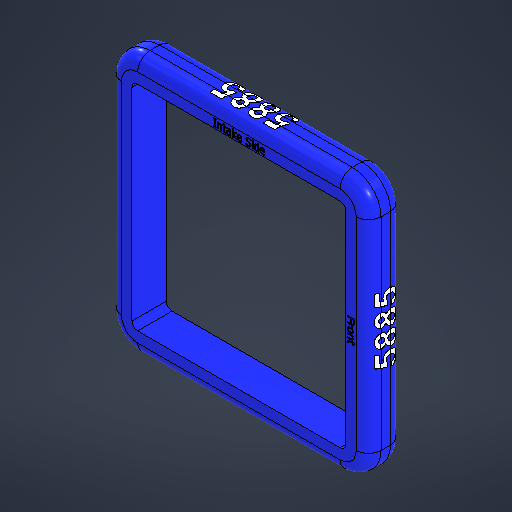
# Autodesk Inventor part: Bumpers
Saved by Autodesk Inventor 2026.1 (Build 301233020, 233B)
## iProperties
Created: 2026-01-21
Part Number: Bumpers
Material: Spruce
Document SubType Name: Modeling
Designer: Jthib
Mass: 13460.1 g
Surface Area: 12229.9 cm^2
Volume: 33650.4 cm^3
Density: 0.4 g/cm^3
Appearance: Blue - Wall Paint - Glossy
Author: Jthib
Autodesk Inventor part; units mm, degrees
ref_plane "YZ Plane" through (0, 0, 0) normal (1, 0, 0) x (0, 1, 0)
ref_plane "XZ Plane" through (0, 0, 0) normal (0, 1, 0) x (-1, 0, 0)
ref_plane "XY Plane" through (0, 0, 0) normal (0, 0, 1) x (1, 0, 0)
sketch "Sketch1" plane through (0, 0, 0) normal (0, 0, 1) x (1, 0, 0)
  line L0 (-349.25, 0) -> (-349.25, 336.55)
  line L1 (-336.55, 349.25) -> (336.55, 349.25)
  line L2 (349.25, 336.55) -> (349.25, -336.55)
  line L3 (336.55, -349.25) -> (-336.55, -349.25)
  line L4 (-349.25, -336.55) -> (-349.25, 0)
  arc A0 (-336.55, 349.25) -> (-349.25, 336.55) centre (-336.55, 336.55) ccw
  arc A1 (349.25, 336.55) -> (336.55, 349.25) centre (336.55, 336.55) ccw
  arc A2 (336.55, -349.25) -> (349.25, -336.55) centre (336.55, -336.55) ccw
  arc A3 (-349.25, -336.55) -> (-336.55, -349.25) centre (-336.55, -336.55) ccw
  point P0 (0, 0)
  point P1 (-349.25, 349.25)
  point P2 (349.25, 349.25)
  point P3 (349.25, -349.25)
  point P4 (-349.25, -349.25)
  dimension "d0" = 698.5
  dimension "d1" = 698.5
  dimension "d2" = 349.25
  dimension "d3" = 349.25
  dimension "d9" = 12.7
  constraints: 10 end point, 9 point on line, 8 point on circle, 8 tangent, 4 centre point, 4 perpendicular, 3 equal radius, 1 collinear, 1 vertical
  measures "d0" distance of point (349.25, 349.25) point (349.25, -349.25)
  measures "d1" distance of point (-349.25, 349.25) point (349.25, 349.25)
  measures "d2" distance from line of point (0, 0) L1
  measures "d3" distance from line of L2 point (0, 0)
  measures "d9" radius of A0
sketch "Sketch2" plane through (0, 0, 0) normal (0, 1, 0) x (-1, 0, 0)
  line L0 (390.525, 61.9125) -> (355.6, 61.9125)
  line L1 (355.6, 61.9125) -> (355.6, -52.3875)
  line L2 (355.6, -52.3875) -> (390.525, -52.3875)
  line L3 (431.8, -11.1125) -> (431.8, 20.6375)
  arc A0 (431.8, 20.6375) -> (390.525, 61.9125) centre (390.525, 20.6375) ccw
  arc A1 (390.525, -52.3875) -> (431.8, -11.1125) centre (390.525, -11.1125) ccw
  line L4 (0, -145.5372) -> (0, 106.4605) construction
  line L5 (355.6, 61.9125) -> (0, 61.9125) construction
  line L6 (355.6, -52.3875) -> (0, -52.3875) construction
  line L7 (-599.1936, -109.5375) -> (599.1891, -109.5375) construction
  point P0 (0, 0)
  point P1 (431.8, 61.9125)
  point P2 (349.25, 0)
  point P3 (349.25, 0)
  point P4 (355.6, 4.7625)
  dimension "d4" = 114.3
  dimension "d5" = 76.2
  dimension "d6" = 41.275
  dimension "d20" = 355.6
  dimension "d21" = 57.15
  constraints: 14 end point, 4 point on circle, 4 point on line, 4 tangent, 3 perpendicular, 2 centre point, 2 horizontal, 2 parallel, 1 equal radius, 1 midpoint, 2 other
  measures "d4" distance of L0.end L1.end
  measures "d5" distance of point (431.8, 61.913) L0.end
  measures "d6" radius of A0
  measures "d20" distance from line of point (0, 0) L1
  measures "d21" distance between parallel lines of L7 L2
sweep "Sweep1" add profiles "Sketch2" path "Sketch1" path curves L0 A0 L1 A1 L2 A2 L3 A3 L4
sketch "Sketch3" plane through (431.8, -336.55, 20.6375) normal (1, 0, 0) x (0, 0, -1)
  line L0 (-23.8125, 82.55) -> (-23.8125, 590.55) construction
  line L1 (-23.8125, 590.55) -> (65.0875, 590.55) construction
  line L2 (65.0875, 590.55) -> (65.0875, 82.55) construction
  line L3 (65.0875, 82.55) -> (-23.8125, 82.55) construction
  line L4 (-23.8125, 82.55) -> (65.0875, 590.55) construction
  line L5 (36.377, 224.9216) -> (35.0992, 239.4995)
  spline S0 degree 2 poles (35.0992, 239.4995) (36.1447, 239.4415) (36.6674, 239.4415) knots 0 0 0 1 1 1
  spline S1 degree 2 poles (36.6674, 239.4415) (41.9526, 239.4415) (47.2378, 244.1459) (47.2378, 247.921) knots 0 0 0 1 2 2 2
  spline S2 degree 2 poles (47.2378, 247.921) (47.2378, 253.2063) (37.132, 261.8601) (28.1878, 261.8601) knots 0 0 0 1 2 2 2
  spline S3 degree 2 poles (28.1878, 261.8601) (22.9026, 261.8601) (17.5012, 256.9814) (17.5012, 252.9159) knots 0 0 0 1 2 2 2
  spline S4 degree 2 poles (17.5012, 252.9159) (17.5012, 250.0119) (20.2309, 244.5524) (22.9607, 241.997) knots 0 0 0 1 2 2 2
  line L6 (22.9607, 241.997) -> (22.0314, 229.7422)
  line L7 (22.0314, 229.7422) -> (-16.9398, 241.3581)
  line L8 (-16.9398, 241.3581) -> (-16.9398, 279.6323)
  line L9 (-16.9398, 279.6323) -> (-3.2912, 276.8445)
  line L10 (-3.2912, 276.8445) -> (-3.2912, 251.522)
  line L11 (-3.2912, 251.522) -> (8.4409, 248.0372)
  spline S5 degree 2 poles (8.4409, 248.0372) (7.4535, 250.2442) (6.4662, 254.6002) (6.4662, 256.7491) knots 0 0 0 1 2 2 2
  spline S6 degree 2 poles (6.4662, 256.7491) (6.4662, 265.461) (18.1982, 276.6703) (28.0716, 276.6703) knots 0 0 0 1 2 2 2
  spline S7 degree 2 poles (28.0716, 276.6703) (35.9704, 276.6703) (51.3034, 268.8296) (59.4925, 254.8906) (59.4925, 247.2822) knots 0 0 0 1 2 3 3 3
  spline S8 degree 2 poles (59.4925, 247.2822) (59.4925, 237.5249) (46.9474, 225.0378) (36.377, 224.9216) knots 0 0 0 1 2 2 2
  spline S9 degree 2 poles (16.2816, 300.2505) (13.668, 296.243) (6.6985, 292.2355) (2.5168, 292.2355) knots 0 0 0 1 2 2 2
  spline S10 degree 2 poles (2.5168, 292.2355) (-2.42, 292.2355) (-12.5258, 297.8692) (-18.3337, 309.0204) (-18.3337, 316.1061) knots 0 0 0 1 2 3 3 3
  spline S11 degree 2 poles (-18.3337, 316.1061) (-18.3337, 326.27) (-7.7052, 337.7116) (0.4259, 337.7116) knots 0 0 0 1 2 2 2
  spline S12 degree 2 poles (0.4259, 337.7116) (6.1177, 337.7116) (14.6553, 331.2648) (17.4431, 324.818) knots 0 0 0 1 2 2 2
  spline S13 degree 2 poles (17.4431, 324.818) (20.289, 329.4643) (28.4782, 334.1107) (33.7053, 334.1107) knots 0 0 0 1 2 2 2
  spline S14 degree 2 poles (33.7053, 334.1107) (42.3591, 334.1107) (49.4448, 328.5931) knots 0 0 0 1 1 1
  spline S15 degree 2 poles (49.4448, 328.5931) (59.6087, 320.5782) (59.6087, 306.7553) knots 0 0 0 1 1 1
  spline S16 degree 2 poles (59.6087, 306.7553) (59.6087, 296.6495) (47.7024, 284.3948) (38.5259, 284.3948) knots 0 0 0 1 2 2 2
  spline S17 degree 2 poles (38.5259, 284.3948) (30.8595, 284.3948) (18.779, 292.9325) (16.2816, 300.2505) knots 0 0 0 1 2 2 2
  spline S18 degree 2 poles (38.7582, 299.2631) (43.0561, 299.2631) (47.9348, 303.9095) (47.9348, 307.6846) knots 0 0 0 1 2 2 2
  spline S19 degree 2 poles (47.9348, 307.6846) (47.9348, 313.4345) (37.7128, 319.707) (31.7306, 319.707) knots 0 0 0 1 2 2 2
  spline S20 degree 2 poles (31.7306, 319.707) (27.8974, 319.707) (22.9607, 314.8864) (22.9607, 311.1694) knots 0 0 0 1 2 2 2
  spline S21 degree 2 poles (22.9607, 311.1694) (22.9607, 306.4649) (31.6145, 299.2631) (38.7582, 299.2631) knots 0 0 0 1 2 2 2
  spline S22 degree 2 poles (3.5041, 305.8841) (7.105, 305.8841) (11.5191, 310.2401) (11.5191, 313.7248) knots 0 0 0 1 2 2 2
  spline S23 degree 2 poles (11.5191, 313.7248) (11.5191, 317.7323) (5.4207, 323.8306) (1.3552, 323.8306) knots 0 0 0 1 2 2 2
  spline S24 degree 2 poles (1.3552, 323.8306) (-2.3038, 323.8306) (-6.8921, 319.3585) (-6.8921, 315.8738) knots 0 0 0 1 2 2 2
  spline S25 degree 2 poles (-6.8921, 315.8738) (-6.8921, 311.7502) (-0.8518, 305.8841) (3.5041, 305.8841) knots 0 0 0 1 2 2 2
  spline S26 degree 2 poles (16.2816, 359.4332) (13.668, 355.4258) (6.6985, 351.4183) (2.5168, 351.4183) knots 0 0 0 1 2 2 2
  spline S27 degree 2 poles (2.5168, 351.4183) (-2.42, 351.4183) (-12.5258, 357.052) (-18.3337, 368.2032) (-18.3337, 375.2889) knots 0 0 0 1 2 3 3 3
  spline S28 degree 2 poles (-18.3337, 375.2889) (-18.3337, 385.4527) (-7.7052, 396.8944) (0.4259, 396.8944) knots 0 0 0 1 2 2 2
  spline S29 degree 2 poles (0.4259, 396.8944) (6.1177, 396.8944) (14.6553, 390.4476) (17.4431, 384.0008) knots 0 0 0 1 2 2 2
  spline S30 degree 2 poles (17.4431, 384.0008) (20.289, 388.6471) (28.4782, 393.2934) (33.7053, 393.2934) knots 0 0 0 1 2 2 2
  spline S31 degree 2 poles (33.7053, 393.2934) (42.3591, 393.2934) (49.4448, 387.7759) knots 0 0 0 1 1 1
  spline S32 degree 2 poles (49.4448, 387.7759) (59.6087, 379.761) (59.6087, 365.9381) knots 0 0 0 1 1 1
  spline S33 degree 2 poles (59.6087, 365.9381) (59.6087, 355.8323) (47.7024, 343.5776) (38.5259, 343.5776) knots 0 0 0 1 2 2 2
  spline S34 degree 2 poles (38.5259, 343.5776) (30.8595, 343.5776) (18.779, 352.1152) (16.2816, 359.4332) knots 0 0 0 1 2 2 2
  spline S35 degree 2 poles (38.7582, 358.4459) (43.0561, 358.4459) (47.9348, 363.0922) (47.9348, 366.8674) knots 0 0 0 1 2 2 2
  spline S36 degree 2 poles (47.9348, 366.8674) (47.9348, 372.6172) (37.7128, 378.8898) (31.7306, 378.8898) knots 0 0 0 1 2 2 2
  spline S37 degree 2 poles (31.7306, 378.8898) (27.8974, 378.8898) (22.9607, 374.0692) (22.9607, 370.3521) knots 0 0 0 1 2 2 2
  spline S38 degree 2 poles (22.9607, 370.3521) (22.9607, 365.6477) (31.6145, 358.4459) (38.7582, 358.4459) knots 0 0 0 1 2 2 2
  spline S39 degree 2 poles (3.5041, 365.0669) (7.105, 365.0669) (11.5191, 369.4229) (11.5191, 372.9076) knots 0 0 0 1 2 2 2
  spline S40 degree 2 poles (11.5191, 372.9076) (11.5191, 376.9151) (5.4207, 383.0134) (1.3552, 383.0134) knots 0 0 0 1 2 2 2
  spline S41 degree 2 poles (1.3552, 383.0134) (-2.3038, 383.0134) (-6.8921, 378.5413) (-6.8921, 375.0566) knots 0 0 0 1 2 2 2
  spline S42 degree 2 poles (-6.8921, 375.0566) (-6.8921, 370.9329) (-0.8518, 365.0669) (3.5041, 365.0669) knots 0 0 0 1 2 2 2
  line L12 (36.377, 402.47) -> (35.0992, 417.0479)
  spline S43 degree 2 poles (35.0992, 417.0479) (36.1447, 416.9898) (36.6674, 416.9898) knots 0 0 0 1 1 1
  spline S44 degree 2 poles (36.6674, 416.9898) (41.9526, 416.9898) (47.2378, 421.6942) (47.2378, 425.4694) knots 0 0 0 1 2 2 2
  spline S45 degree 2 poles (47.2378, 425.4694) (47.2378, 430.7546) (37.132, 439.4084) (28.1878, 439.4084) knots 0 0 0 1 2 2 2
  spline S46 degree 2 poles (28.1878, 439.4084) (22.9026, 439.4084) (17.5012, 434.5297) (17.5012, 430.4642) knots 0 0 0 1 2 2 2
  spline S47 degree 2 poles (17.5012, 430.4642) (17.5012, 427.5602) (20.2309, 422.1008) (22.9607, 419.5453) knots 0 0 0 1 2 2 2
  line L13 (22.9607, 419.5453) -> (22.0314, 407.2905)
  line L14 (22.0314, 407.2905) -> (-16.9398, 418.9064)
  line L15 (-16.9398, 418.9064) -> (-16.9398, 457.1806)
  line L16 (-16.9398, 457.1806) -> (-3.2912, 454.3928)
  line L17 (-3.2912, 454.3928) -> (-3.2912, 429.0703)
  line L18 (-3.2912, 429.0703) -> (8.4409, 425.5855)
  spline S48 degree 2 poles (8.4409, 425.5855) (7.4535, 427.7925) (6.4662, 432.1485) (6.4662, 434.2974) knots 0 0 0 1 2 2 2
  spline S49 degree 2 poles (6.4662, 434.2974) (6.4662, 443.0093) (18.1982, 454.2186) (28.0716, 454.2186) knots 0 0 0 1 2 2 2
  spline S50 degree 2 poles (28.0716, 454.2186) (35.9704, 454.2186) (51.3034, 446.3779) (59.4925, 432.4389) (59.4925, 424.8305) knots 0 0 0 1 2 3 3 3
  spline S51 degree 2 poles (59.4925, 424.8305) (59.4925, 415.0732) (46.9474, 402.5861) (36.377, 402.47) knots 0 0 0 1 2 2 2
  point P0 (20.6375, 336.55)
  point P1 (20.6375, 336.55)
  dimension "d2" = 349.25
  dimension "d10" = 508
  dimension "d11" = 88.9
  constraints: 2 end point, 1 coincident, 1 horizontal, 1 midpoint, 2 other
  measures "d10" distance of L0.start L0.end
  measures "d11" distance of L0.end L1.end
emboss "Emboss1" sketch "Sketch3" operation cut depth 0.254 direction (-1, 0, 0)
pattern_circular "Circular Pattern1" count 4 over 360 about axis through (0, 0, -10) along (0, 0, 1) of "Emboss1"
sketch "Sketch4" plane through (-336.55, -390.525, 61.9125) normal (0, 0, 1) x (1, 0, 0)
  line L0 (692.15, 517.525) -> (692.15, 263.525) construction
  line L1 (692.15, 263.525) -> (727.075, 263.525) construction
  line L2 (727.075, 263.525) -> (727.075, 517.525) construction
  line L3 (727.075, 517.525) -> (692.15, 517.525) construction
  line L4 (692.15, 727.075) -> (692.15, 53.975) projected
  line L5 (727.075, 727.075) -> (727.075, 53.975) projected
  line L6 (719.5749, 413.2286) -> (719.5749, 425.0435)
  line L7 (719.5749, 425.0435) -> (712.4119, 425.0435)
  line L8 (712.4119, 425.0435) -> (712.4119, 413.7226)
  line L9 (712.4119, 413.7226) -> (709.4067, 413.7226)
  line L10 (709.4067, 413.7226) -> (709.4067, 425.0435)
  line L11 (709.4067, 425.0435) -> (697.1801, 425.0435)
  line L12 (697.1801, 425.0435) -> (697.1801, 428.4192)
  line L13 (697.1801, 428.4192) -> (722.5801, 428.4192)
  line L14 (722.5801, 428.4192) -> (722.5801, 413.2286)
  line L15 (722.5801, 413.2286) -> (719.5749, 413.2286)
  line L16 (712.8029, 400.3433) -> (712.8029, 400.508)
  spline S0 degree 2 poles (712.8029, 400.508) (712.9059, 400.8785) (712.947, 401.6812) (712.947, 402.237) knots 0 0 0 1 2 2 2
  spline S1 degree 2 poles (712.947, 402.237) (712.947, 403.5337) (711.8149, 406.0861) (710.7034, 407.2388) knots 0 0 0 1 2 2 2
  line L17 (710.7034, 407.2388) -> (697.1801, 407.2388)
  line L18 (697.1801, 407.2388) -> (697.1801, 410.4498)
  line L19 (697.1801, 410.4498) -> (716.2404, 410.4498)
  line L20 (716.2404, 410.4498) -> (716.2404, 407.2388)
  line L21 (716.2404, 407.2388) -> (713.3999, 407.2388)
  spline S2 degree 2 poles (713.3999, 407.2388) (714.9642, 405.4892) (716.2404, 402.8751) (716.2404, 401.6401) knots 0 0 0 1 2 2 2
  spline S3 degree 2 poles (716.2404, 401.6401) (716.2404, 401.1461) (716.1992, 400.6521) (716.1375, 400.3433) knots 0 0 0 1 2 2 2
  line L22 (716.1375, 400.3433) -> (712.8029, 400.3433)
  spline S4 degree 2 poles (706.7102, 382.1887) (701.8937, 382.1887) (696.6449, 386.82) (696.6449, 390.6897) knots 0 0 0 1 2 2 2
  spline S5 degree 2 poles (696.6449, 390.6897) (696.6449, 394.6623) (702.0584, 399.2112) (706.7102, 399.2112) knots 0 0 0 1 2 2 2
  spline S6 degree 2 poles (706.7102, 399.2112) (711.4856, 399.2112) (716.7755, 394.5182) (716.7755, 390.6897) knots 0 0 0 1 2 2 2
  spline S7 degree 2 poles (716.7755, 390.6897) (716.7755, 386.82) (711.5062, 382.1887) (706.7102, 382.1887) knots 0 0 0 1 2 2 2
  spline S8 degree 2 poles (706.7102, 385.5026) (710.4153, 385.5026) (714.0174, 388.1991) (714.0174, 390.6897) knots 0 0 0 1 2 2 2
  spline S9 degree 2 poles (714.0174, 390.6897) (714.0174, 393.1803) (710.4153, 395.8973) (706.7102, 395.8973) knots 0 0 0 1 2 2 2
  spline S10 degree 2 poles (706.7102, 395.8973) (703.1081, 395.8973) (699.4031, 393.1803) (699.4031, 390.6897) knots 0 0 0 1 2 2 2
  spline S11 degree 2 poles (699.4031, 390.6897) (699.4031, 388.2196) (703.0464, 385.5026) (706.7102, 385.5026) knots 0 0 0 1 2 2 2
  line L23 (697.1801, 363.9312) -> (697.1801, 367.1422)
  line L24 (697.1801, 367.1422) -> (708.0482, 367.1422)
  spline S12 degree 2 poles (708.0482, 367.1422) (709.3655, 367.1422) (711.6297, 367.3892) (712.3089, 367.7597) knots 0 0 0 1 2 2 2
  spline S13 degree 2 poles (712.3089, 367.7597) (713.0294, 368.1508) (713.7292, 369.5504) (713.7292, 370.7443) knots 0 0 0 1 2 2 2
  spline S14 degree 2 poles (713.7292, 370.7443) (713.7292, 371.9381) (712.453, 374.4699) (711.4238, 375.6843) knots 0 0 0 1 2 2 2
  line L25 (711.4238, 375.6843) -> (697.1801, 375.6843)
  line L26 (697.1801, 375.6843) -> (697.1801, 378.8953)
  line L27 (697.1801, 378.8953) -> (716.2404, 378.8953)
  line L28 (716.2404, 378.8953) -> (716.2404, 375.6843)
  line L29 (716.2404, 375.6843) -> (714.1203, 375.6843)
  spline S15 degree 2 poles (714.1203, 375.6843) (715.417, 374.2435) (716.7755, 371.4647) (716.7755, 369.9004) knots 0 0 0 1 2 2 2
  spline S16 degree 2 poles (716.7755, 369.9004) (716.7755, 367.101) (713.0705, 363.9312) (709.5507, 363.9312) knots 0 0 0 1 2 2 2
  line L30 (709.5507, 363.9312) -> (697.1801, 363.9312)
  spline S17 degree 2 poles (696.8096, 353.66) (696.8096, 356.2741) (699.7942, 359.2175) (703.0258, 359.2175) knots 0 0 0 1 2 2 2
  line L31 (703.0258, 359.2175) -> (713.5851, 359.2175)
  line L32 (713.5851, 359.2175) -> (713.5851, 361.3788)
  line L33 (713.5851, 361.3788) -> (716.2404, 361.3788)
  line L34 (716.2404, 361.3788) -> (716.2404, 359.2175)
  line L35 (716.2404, 359.2175) -> (721.7156, 359.2175)
  line L36 (721.7156, 359.2175) -> (721.7156, 356.0065)
  line L37 (721.7156, 356.0065) -> (716.2404, 356.0065)
  line L38 (716.2404, 356.0065) -> (716.2404, 350.0991)
  line L39 (716.2404, 350.0991) -> (713.5851, 350.0991)
  line L40 (713.5851, 350.0991) -> (713.5851, 356.0065)
  line L41 (713.5851, 356.0065) -> (704.5078, 356.0065)
  spline S18 degree 2 poles (704.5078, 356.0065) (703.067, 356.0065) (701.482, 355.9036) (700.8028, 355.5537) knots 0 0 0 1 2 2 2
  spline S19 degree 2 poles (700.8028, 355.5537) (700.2059, 355.2655) (699.6089, 353.9688) (699.6089, 352.8573) knots 0 0 0 1 2 2 2
  spline S20 degree 2 poles (699.6089, 352.8573) (699.6089, 352.0751) (700.0824, 350.6137) (700.2264, 350.2843) knots 0 0 0 1 2 2 2
  line L42 (700.2264, 350.2843) -> (700.2264, 350.0991)
  line L43 (700.2264, 350.0991) -> (697.3448, 350.0991)
  spline S21 degree 2 poles (697.3448, 350.0991) (697.0978, 351.0047) (696.8096, 352.8573) (696.8096, 353.66) knots 0 0 0 1 2 2 2
  point P0 (336.55, 390.525)
  point P1 (727.075, 390.525)
  dimension "d2" = 349.25
  dimension "d17" = 254
  constraints: 2 midpoint, 1 collinear, 2 other
  measures "d17" distance between parallel lines of L1 L3
emboss "Emboss2" sketch "Sketch4" operation cut depth 0.254 direction (0, 0, -1)
sketch "Sketch5" plane through (-336.55, -390.525, 61.9125) normal (0, 0, 1) x (1, 0, 0)
  line L0 (0, 781.05) -> (673.1, 781.05) construction
  line L1 (673.1, 781.05) -> (673.1, 746.125) construction
  line L2 (673.1, 746.125) -> (0, 746.125) construction
  line L3 (0, 746.125) -> (0, 781.05) construction
  line L4 (0, 781.05) -> (673.1, 781.05) construction
  line L5 (0, 746.125) -> (673.1, 746.125) construction
  line L6 (336.55, -215.9) -> (336.55, 1006.475) construction
  line L7 (260.8028, 750.589) -> (250.9639, 750.589)
  line L8 (250.9639, 750.589) -> (250.9639, 753.1826)
  line L9 (250.9639, 753.1826) -> (254.1955, 753.1826)
  line L10 (254.1955, 753.1826) -> (254.1955, 773.3955)
  line L11 (254.1955, 773.3955) -> (250.9639, 773.3955)
  line L12 (250.9639, 773.3955) -> (250.9639, 775.989)
  line L13 (250.9639, 775.989) -> (260.8028, 775.989)
  line L14 (260.8028, 775.989) -> (260.8028, 773.3955)
  line L15 (260.8028, 773.3955) -> (257.5712, 773.3955)
  line L16 (257.5712, 773.3955) -> (257.5712, 753.1826)
  line L17 (257.5712, 753.1826) -> (260.8028, 753.1826)
  line L18 (260.8028, 753.1826) -> (260.8028, 750.589)
  line L19 (279.6985, 750.589) -> (276.4874, 750.589)
  line L20 (276.4874, 750.589) -> (276.4874, 761.4571)
  spline S0 degree 2 poles (276.4874, 761.4571) (276.4874, 762.7745) (276.2404, 765.0386) (275.8699, 765.7179) knots 0 0 0 1 2 2 2
  spline S1 degree 2 poles (275.8699, 765.7179) (275.4789, 766.4383) (274.0792, 767.1381) (272.8853, 767.1381) knots 0 0 0 1 2 2 2
  spline S2 degree 2 poles (272.8853, 767.1381) (271.6915, 767.1381) (269.1597, 765.862) (267.9453, 764.8328) knots 0 0 0 1 2 2 2
  line L21 (267.9453, 764.8328) -> (267.9453, 750.589)
  line L22 (267.9453, 750.589) -> (264.7343, 750.589)
  line L23 (264.7343, 750.589) -> (264.7343, 769.6493)
  line L24 (264.7343, 769.6493) -> (267.9453, 769.6493)
  line L25 (267.9453, 769.6493) -> (267.9453, 767.5292)
  spline S3 degree 2 poles (267.9453, 767.5292) (269.3861, 768.826) (272.1649, 770.1845) (273.7293, 770.1845) knots 0 0 0 1 2 2 2
  spline S4 degree 2 poles (273.7293, 770.1845) (276.5286, 770.1845) (279.6985, 766.4795) (279.6985, 762.9597) knots 0 0 0 1 2 2 2
  line L26 (279.6985, 762.9597) -> (279.6985, 750.589)
  spline S5 degree 2 poles (289.9696, 750.2185) (287.3555, 750.2185) (284.4121, 753.2031) (284.4121, 756.4347) knots 0 0 0 1 2 2 2
  line L27 (284.4121, 756.4347) -> (284.4121, 766.9941)
  line L28 (284.4121, 766.9941) -> (282.2508, 766.9941)
  line L29 (282.2508, 766.9941) -> (282.2508, 769.6493)
  line L30 (282.2508, 769.6493) -> (284.4121, 769.6493)
  line L31 (284.4121, 769.6493) -> (284.4121, 775.1245)
  line L32 (284.4121, 775.1245) -> (287.6231, 775.1245)
  line L33 (287.6231, 775.1245) -> (287.6231, 769.6493)
  line L34 (287.6231, 769.6493) -> (293.5306, 769.6493)
  line L35 (293.5306, 769.6493) -> (293.5306, 766.9941)
  line L36 (293.5306, 766.9941) -> (287.6231, 766.9941)
  line L37 (287.6231, 766.9941) -> (287.6231, 757.9168)
  spline S6 degree 2 poles (287.6231, 757.9168) (287.6231, 756.4759) (287.726, 754.891) (288.0759, 754.2117) knots 0 0 0 1 2 2 2
  spline S7 degree 2 poles (288.0759, 754.2117) (288.3641, 753.6148) (289.6609, 753.0179) (290.7724, 753.0179) knots 0 0 0 1 2 2 2
  spline S8 degree 2 poles (290.7724, 753.0179) (291.5545, 753.0179) (293.016, 753.4913) (293.3453, 753.6354) knots 0 0 0 1 2 2 2
  line L38 (293.3453, 753.6354) -> (293.5306, 753.6354)
  line L39 (293.5306, 753.6354) -> (293.5306, 750.7537)
  spline S9 degree 2 poles (293.5306, 750.7537) (292.6249, 750.5067) (290.7724, 750.2185) (289.9696, 750.2185) knots 0 0 0 1 2 2 2
  spline S10 degree 2 poles (306.5187, 752.6062) (306.1276, 752.3181) (304.8103, 751.2889) (304.1928, 750.9801) knots 0 0 0 1 2 2 2
  spline S11 degree 2 poles (304.1928, 750.9801) (303.3489, 750.5273) (301.7639, 750.0539) (300.3231, 750.0539) knots 0 0 0 1 2 2 2
  spline S12 degree 2 poles (300.3231, 750.0539) (299.1498, 750.0539) (297.0297, 750.939) (296.227, 751.7417) knots 0 0 0 1 2 2 2
  spline S13 degree 2 poles (296.227, 751.7417) (295.4654, 752.5239) (294.5391, 754.8292) (294.5391, 756.1054) knots 0 0 0 1 2 2 2
  spline S14 degree 2 poles (294.5391, 756.1054) (294.5391, 758.0814) (296.2064, 760.8808) (298.0178, 761.6835) knots 0 0 0 1 2 2 2
  spline S15 degree 2 poles (298.0178, 761.6835) (299.6233, 762.4245) (303.987, 762.9803) (306.5187, 763.1244) knots 0 0 0 1 2 2 2
  line L40 (306.5187, 763.1244) -> (306.5187, 763.7419)
  spline S16 degree 2 poles (306.5187, 763.7419) (306.5187, 764.8534) (305.8395, 766.2325) (305.222, 766.6236) knots 0 0 0 1 2 2 2
  spline S17 degree 2 poles (305.222, 766.6236) (304.6045, 767.0146) (302.8343, 767.2616) (301.8874, 767.2616) knots 0 0 0 1 2 2 2
  spline S18 degree 2 poles (301.8874, 767.2616) (300.7759, 767.2616) (297.7708, 766.603) (296.2682, 765.9649) knots 0 0 0 1 2 2 2
  line L41 (296.2682, 765.9649) -> (296.0829, 765.9649)
  line L42 (296.0829, 765.9649) -> (296.0829, 769.2377)
  spline S19 degree 2 poles (296.0829, 769.2377) (296.968, 769.4847) (300.2819, 770.1022) (301.908, 770.1022) knots 0 0 0 1 2 2 2
  spline S20 degree 2 poles (301.908, 770.1022) (303.884, 770.1022) (306.5805, 769.4847) (307.6508, 768.6819) knots 0 0 0 1 2 2 2
  spline S21 degree 2 poles (307.6508, 768.6819) (308.7006, 767.8997) (309.7297, 765.4091) (309.7297, 763.6184) knots 0 0 0 1 2 2 2
  line L43 (309.7297, 763.6184) -> (309.7297, 750.589)
  line L44 (309.7297, 750.589) -> (306.5187, 750.589)
  line L45 (306.5187, 750.589) -> (306.5187, 752.6062)
  line L46 (306.5187, 755.2821) -> (306.5187, 760.572)
  spline S22 degree 2 poles (306.5187, 760.572) (305.3661, 760.4691) (301.8874, 760.1192) (300.7965, 759.7899) knots 0 0 0 1 2 2 2
  spline S23 degree 2 poles (300.7965, 759.7899) (299.5203, 759.3988) (297.8531, 757.7727) (297.8531, 756.3318) knots 0 0 0 1 2 2 2
  spline S24 degree 2 poles (297.8531, 756.3318) (297.8531, 754.6852) (299.7056, 753.0179) (301.4758, 753.0179) knots 0 0 0 1 2 2 2
  spline S25 degree 2 poles (301.4758, 753.0179) (302.9784, 753.0179) (305.4484, 754.3146) (306.5187, 755.2821) knots 0 0 0 1 2 2 2
  line L47 (330.025, 750.589) -> (325.8054, 750.589)
  line L48 (325.8054, 750.589) -> (318.7247, 759.7899)
  line L49 (318.7247, 759.7899) -> (317.4485, 758.5548)
  line L50 (317.4485, 758.5548) -> (317.4485, 750.589)
  line L51 (317.4485, 750.589) -> (314.2375, 750.589)
  line L52 (314.2375, 750.589) -> (314.2375, 777.1211)
  line L53 (314.2375, 777.1211) -> (317.4485, 777.1211)
  line L54 (317.4485, 777.1211) -> (317.4485, 761.6012)
  line L55 (317.4485, 761.6012) -> (324.9821, 769.6493)
  line L56 (324.9821, 769.6493) -> (328.9753, 769.6493)
  line L57 (328.9753, 769.6493) -> (321.1536, 761.6835)
  line L58 (321.1536, 761.6835) -> (330.025, 750.589)
  spline S26 degree 2 poles (339.9051, 750.1568) (335.3356, 750.1568) (330.3132, 755.2821) (330.3132, 760.0163) knots 0 0 0 1 2 2 2
  spline S27 degree 2 poles (330.3132, 760.0163) (330.3132, 764.6681) (335.1915, 770.1845) (339.1229, 770.1845) knots 0 0 0 1 2 2 2
  spline S28 degree 2 poles (339.1229, 770.1845) (340.8931, 770.1845) (343.6307, 769.1553) (344.6393, 768.0644) knots 0 0 0 1 2 2 2
  spline S29 degree 2 poles (344.6393, 768.0644) (345.6685, 766.9735) (346.7594, 763.8242) (346.7594, 761.5394) knots 0 0 0 1 2 2 2
  line L59 (346.7594, 761.5394) -> (346.7594, 759.7899)
  line L60 (346.7594, 759.7899) -> (333.5654, 759.7899)
  spline S30 degree 2 poles (333.5654, 759.7899) (333.5654, 756.4759) (336.8999, 752.9561) (339.8639, 752.9561) knots 0 0 0 1 2 2 2
  spline S31 degree 2 poles (339.8639, 752.9561) (340.9137, 752.9561) (342.9515, 753.4296) (343.7748, 753.8001) knots 0 0 0 1 2 2 2
  spline S32 degree 2 poles (343.7748, 753.8001) (344.6393, 754.2117) (345.8331, 754.9322) (346.2242, 755.2615) knots 0 0 0 1 2 2 2
  line L61 (346.2242, 755.2615) -> (346.4095, 755.2615)
  line L62 (346.4095, 755.2615) -> (346.4095, 751.7623)
  spline S33 degree 2 poles (346.4095, 751.7623) (345.8537, 751.5359) (344.1659, 750.8772) (343.5072, 750.692) knots 0 0 0 1 2 2 2
  spline S34 degree 2 poles (343.5072, 750.692) (342.581, 750.4244) (341.0578, 750.1568) (339.9051, 750.1568) knots 0 0 0 1 2 2 2
  spline S35 degree 2 poles (343.6307, 762.2393) (343.5896, 763.536) (343.0544, 765.4297) (342.5398, 766.0678) knots 0 0 0 1 2 2 2
  spline S36 degree 2 poles (342.5398, 766.0678) (341.984, 766.7882) (340.2344, 767.5498) (338.9377, 767.5498) knots 0 0 0 1 2 2 2
  spline S37 degree 2 poles (338.9377, 767.5498) (337.6615, 767.5498) (335.8708, 766.7882) (335.1297, 766.0472) knots 0 0 0 1 2 2 2
  spline S38 degree 2 poles (335.1297, 766.0472) (334.4093, 765.2856) (333.6683, 763.4537) (333.5654, 762.2393) knots 0 0 0 1 2 2 2
  line L63 (333.5654, 762.2393) -> (343.6307, 762.2393)
  spline S39 degree 2 poles (368.2485, 750.1362) (365.4904, 750.1362) (361.6207, 751.2889) (359.9122, 752.1122) knots 0 0 0 1 2 2 2
  line L64 (359.9122, 752.1122) -> (359.9122, 756.3524)
  line L65 (359.9122, 756.3524) -> (360.1592, 756.3524)
  spline S40 degree 2 poles (360.1592, 756.3524) (361.8265, 754.7881) (366.0461, 753.0591) (368.0015, 753.0591) knots 0 0 0 1 2 2 2
  spline S41 degree 2 poles (368.0015, 753.0591) (370.8009, 753.0591) (373.662, 755.385) (373.662, 757.2993) knots 0 0 0 1 2 2 2
  spline S42 degree 2 poles (373.662, 757.2993) (373.662, 758.8224) (372.1594, 760.7161) (370.5333, 761.1895) knots 0 0 0 1 2 2 2
  spline S43 degree 2 poles (370.5333, 761.1895) (369.3601, 761.5189) (367.4046, 761.9717) (365.9432, 762.3422) knots 0 0 0 1 2 2 2
  spline S44 degree 2 poles (365.9432, 762.3422) (364.6259, 762.6921) (362.5469, 763.7419) (361.7442, 764.5858) knots 0 0 0 1 2 2 2
  spline S45 degree 2 poles (361.7442, 764.5858) (360.962, 765.4297) (360.0975, 767.6939) (360.0975, 769.1759) knots 0 0 0 1 2 2 2
  spline S46 degree 2 poles (360.0975, 769.1759) (360.0975, 772.2634) (364.914, 776.4419) (368.6396, 776.4419) knots 0 0 0 1 2 2 2
  spline S47 degree 2 poles (368.6396, 776.4419) (370.7803, 776.4419) (374.5677, 775.598) (376.1938, 774.7952) knots 0 0 0 1 2 2 2
  line L66 (376.1938, 774.7952) -> (376.1938, 770.7608)
  line L67 (376.1938, 770.7608) -> (375.9468, 770.7608)
  spline S48 degree 2 poles (375.9468, 770.7608) (374.7323, 771.8723) (370.945, 773.519) (368.866, 773.519) knots 0 0 0 1 2 2 2
  spline S49 degree 2 poles (368.866, 773.519) (366.5195, 773.519) (363.6173, 771.3166) (363.6173, 769.5258) knots 0 0 0 1 2 2 2
  spline S50 degree 2 poles (363.6173, 769.5258) (363.6173, 767.9203) (365.3257, 766.0061) (366.9312, 765.5738) knots 0 0 0 1 2 2 2
  spline S51 degree 2 poles (366.9312, 765.5738) (368.0015, 765.2856) (371.1096, 764.5446) (372.1388, 764.2359) knots 0 0 0 1 2 2 2
  spline S52 degree 2 poles (372.1388, 764.2359) (374.7529, 763.4331) (377.1818, 760.2015) (377.1818, 757.8344) knots 0 0 0 1 2 2 2
  spline S53 degree 2 poles (377.1818, 757.8344) (377.1818, 756.3318) (375.9673, 753.4501) (374.8764, 752.4416) knots 0 0 0 1 2 2 2
  spline S54 degree 2 poles (374.8764, 752.4416) (373.662, 751.33) (370.5745, 750.1362) (368.2485, 750.1362) knots 0 0 0 1 2 2 2
  line L68 (383.645, 750.589) -> (380.434, 750.589)
  line L69 (380.434, 750.589) -> (380.434, 769.6493)
  line L70 (380.434, 769.6493) -> (383.645, 769.6493)
  line L71 (383.645, 769.6493) -> (383.645, 750.589)
  line L72 (383.8714, 772.8192) -> (380.2281, 772.8192)
  line L73 (380.2281, 772.8192) -> (380.2281, 776.1537)
  line L74 (380.2281, 776.1537) -> (383.8714, 776.1537)
  line L75 (383.8714, 776.1537) -> (383.8714, 772.8192)
  line L76 (403.014, 750.589) -> (399.803, 750.589)
  line L77 (399.803, 750.589) -> (399.803, 752.5239)
  spline S55 degree 2 poles (399.803, 752.5239) (399.062, 751.9064) (397.9711, 751.083) (397.2301, 750.7331) knots 0 0 0 1 2 2 2
  spline S56 degree 2 poles (397.2301, 750.7331) (396.5508, 750.4038) (395.0894, 750.0539) (394.122, 750.0539) knots 0 0 0 1 2 2 2
  spline S57 degree 2 poles (394.122, 750.0539) (392.5576, 750.0539) (389.9229, 751.3506) (388.9967, 752.6062) knots 0 0 0 1 2 2 2
  spline S58 degree 2 poles (388.9967, 752.6062) (388.0704, 753.8618) (387.0413, 757.5668) (387.0413, 759.9751) knots 0 0 0 1 2 2 2
  spline S59 degree 2 poles (387.0413, 759.9751) (387.0413, 762.4863) (388.338, 766.1501) (389.4701, 767.5292) knots 0 0 0 1 2 2 2
  spline S60 degree 2 poles (389.4701, 767.5292) (390.5199, 768.7642) (393.4633, 770.1845) (395.0894, 770.1845) knots 0 0 0 1 2 2 2
  spline S61 degree 2 poles (395.0894, 770.1845) (396.5096, 770.1845) (398.6297, 769.5464) (399.803, 768.8877) knots 0 0 0 1 2 2 2
  line L78 (399.803, 768.8877) -> (399.803, 777.1211)
  line L79 (399.803, 777.1211) -> (403.014, 777.1211)
  line L80 (403.014, 777.1211) -> (403.014, 750.589)
  line L81 (399.803, 755.2203) -> (399.803, 766.2325)
  spline S62 degree 2 poles (399.803, 766.2325) (398.6092, 766.8088) (396.7155, 767.2411) (395.6246, 767.2411) knots 0 0 0 1 2 2 2
  spline S63 degree 2 poles (395.6246, 767.2411) (393.1545, 767.2411) (390.3552, 763.536) (390.3552, 760.0369) knots 0 0 0 1 2 2 2
  spline S64 degree 2 poles (390.3552, 760.0369) (390.3552, 756.6612) (392.4959, 753.1002) (394.863, 753.1002) knots 0 0 0 1 2 2 2
  spline S65 degree 2 poles (394.863, 753.1002) (396.1186, 753.1002) (398.6709, 754.2529) (399.803, 755.2203) knots 0 0 0 1 2 2 2
  spline S66 degree 2 poles (415.9404, 750.1568) (411.3709, 750.1568) (406.3485, 755.2821) (406.3485, 760.0163) knots 0 0 0 1 2 2 2
  spline S67 degree 2 poles (406.3485, 760.0163) (406.3485, 764.6681) (411.2268, 770.1845) (415.1583, 770.1845) knots 0 0 0 1 2 2 2
  spline S68 degree 2 poles (415.1583, 770.1845) (416.9284, 770.1845) (419.666, 769.1553) (420.6746, 768.0644) knots 0 0 0 1 2 2 2
  spline S69 degree 2 poles (420.6746, 768.0644) (421.7038, 766.9735) (422.7947, 763.8242) (422.7947, 761.5394) knots 0 0 0 1 2 2 2
  line L82 (422.7947, 761.5394) -> (422.7947, 759.7899)
  line L83 (422.7947, 759.7899) -> (409.6007, 759.7899)
  spline S70 degree 2 poles (409.6007, 759.7899) (409.6007, 756.4759) (412.9353, 752.9561) (415.8993, 752.9561) knots 0 0 0 1 2 2 2
  spline S71 degree 2 poles (415.8993, 752.9561) (416.949, 752.9561) (418.9868, 753.4296) (419.8101, 753.8001) knots 0 0 0 1 2 2 2
  spline S72 degree 2 poles (419.8101, 753.8001) (420.6746, 754.2117) (421.8685, 754.9322) (422.2596, 755.2615) knots 0 0 0 1 2 2 2
  line L84 (422.2596, 755.2615) -> (422.4448, 755.2615)
  line L85 (422.4448, 755.2615) -> (422.4448, 751.7623)
  spline S73 degree 2 poles (422.4448, 751.7623) (421.8891, 751.5359) (420.2012, 750.8772) (419.5425, 750.692) knots 0 0 0 1 2 2 2
  spline S74 degree 2 poles (419.5425, 750.692) (418.6163, 750.4244) (417.0931, 750.1568) (415.9404, 750.1568) knots 0 0 0 1 2 2 2
  spline S75 degree 2 poles (419.666, 762.2393) (419.6249, 763.536) (419.0897, 765.4297) (418.5751, 766.0678) knots 0 0 0 1 2 2 2
  spline S76 degree 2 poles (418.5751, 766.0678) (418.0194, 766.7882) (416.2698, 767.5498) (414.973, 767.5498) knots 0 0 0 1 2 2 2
  spline S77 degree 2 poles (414.973, 767.5498) (413.6968, 767.5498) (411.9061, 766.7882) (411.1651, 766.0472) knots 0 0 0 1 2 2 2
  spline S78 degree 2 poles (411.1651, 766.0472) (410.4447, 765.2856) (409.7037, 763.4537) (409.6007, 762.2393) knots 0 0 0 1 2 2 2
  line L86 (409.6007, 762.2393) -> (419.666, 762.2393)
  point P0 (336.55, 390.525)
  point P1 (336.55, 746.125)
  dimension "d2" = 349.25
  constraints: 3 collinear, 1 midpoint, 1 point on line, 2 other
emboss "Emboss3" sketch "Sketch5" operation cut depth 0.254 direction (0, 0, -1)
equation "\"d2\" = 0.5 * d0"
equation "\"d0\" = d1"
equation "\"d3\" = 0.5 * d1"
body "Solid1"
